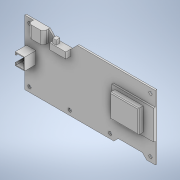
# Autodesk Inventor part: mcu-unit
Saved by Autodesk Inventor 2021 (Build 250183000, 183)
## iProperties
Created: 2024-04-23
Part Number: mcu-unit
Material: Generic
Document SubType Name: Modeling
Designer: Toby
Density: 1 g/cm^3
Appearance: Default
Author: Toby
Autodesk Inventor part; units mm, degrees
ref_plane "YZ Plane" through (0, 0, 0) normal (1, 0, 0) x (0, 1, 0)
ref_plane "XZ Plane" through (0, 0, 0) normal (0, 1, 0) x (-1, 0, 0)
ref_plane "XY Plane" through (0, 0, 0) normal (0, 0, 1) x (1, 0, 0)
sketch "Sketch1" plane through (0, 0, 0) normal (0, 0, 1) x (1, 0, 0)
  line L0 (-40.5, 20) -> (40.5, 20)
  line L1 (40.5, 20) -> (40.5, -20)
  line L2 (40.5, -20) -> (-40.5, -20)
  line L3 (-40.5, -20) -> (-40.5, 20)
  point P0 (0, 0)
  dimension "d0" = 81
  dimension "d1" = 40
  dimension "d2" = 20
  dimension "d3" = 40.5
  constraints: 8 end point, 2 parallel, 1 horizontal, 1 perpendicular
  measures "d0" distance of L0.start L0.end
  measures "d1" distance of L0.end L1.end
  measures "d2" distance from line of point (0, 0) L0
  measures "d3" distance from line of L1 point (0, 0)
extrude "Extrusion1" add sketch "Sketch1" along normal blind 1
sketch "Sketch2" plane through (0, 0, 1) normal (0, 0, 1) x (1, 0, 0)
  line L0 (40.5, 20) -> (-40.5, 20) projected
  line L1 (-21.8, 20) -> (-11.7, 20)
  line L2 (-11.7, 20) -> (-11.7, 16.1)
  line L3 (-11.7, 16.1) -> (-21.8, 16.1)
  line L4 (-21.8, 16.1) -> (-21.8, 20)
  line L5 (-40.5, 20) -> (-40.5, -20) projected
  point P0 (0, 0)
  dimension "d6" = 18.7
  dimension "d7" = 28.8
  dimension "d8" = 3.9
  constraints: 8 end point, 2 parallel, 1 horizontal, 1 perpendicular, 1 point on line
  measures "d6" distance between parallel lines of L5 L4
  measures "d7" distance between parallel lines of L5 L2
  measures "d8" distance between parallel lines of L3 L0
extrude "Extrusion2" cut sketch "Sketch2" against normal blind 1
chamfer "Chamfer1" distance 3.88 angle 45 2 edges at (-21.8, 20, 0.5) (-11.7, 20, 0.5)
sketch "Sketch3" plane through (0, 0, 1) normal (0, 0, 1) x (1, 0, 0)
  line L0 (-25.68, 20) -> (-40.5, 20) projected
  line L1 (-35.04, 20) -> (-25.77, 20)
  line L2 (-25.77, 20) -> (-25.77, 12.38)
  line L3 (-25.77, 12.38) -> (-35.04, 12.38)
  line L4 (-35.04, 12.38) -> (-35.04, 20)
  line L5 (-40.5, 20) -> (-40.5, -20) projected
  point P0 (0, 0)
  dimension "d14" = 5.46
  dimension "d15" = 14.73
  dimension "d16" = 7.62
  constraints: 8 end point, 2 parallel, 1 horizontal, 1 perpendicular, 1 point on line
  measures "d14" distance between parallel lines of L5 L4
  measures "d15" distance between parallel lines of L5 L2
  measures "d16" distance of L3.end L1.start
extrude "Extrusion3" add sketch "Sketch3" along normal blind 3.2
fillet "Fillet1" radius 2 2 edges at (-35.04, 16.19, 4.2) (-25.77, 16.19, 4.2)
sketch "Sketch4" plane through (0, 0, 1) normal (0, 0, 1) x (1, 0, 0)
  line L0 (-11.7, 16.1) -> (-21.8, 16.1) projected
  line L1 (-21.8, 16.1) -> (-11.8, 16.1)
  line L2 (-11.8, 16.1) -> (-11.8, 12.3)
  line L3 (-11.8, 12.3) -> (-21.8, 12.3)
  line L4 (-21.8, 12.3) -> (-21.8, 16.1)
  point P0 (0, 0)
  dimension "d20" = 3.8
  dimension "d21" = 10
  constraints: 8 end point, 2 parallel, 1 horizontal, 1 perpendicular
  measures "d20" distance of L1.end L2.end
  measures "d21" distance between parallel lines of L4 L2
extrude "Extrusion4" add sketch "Sketch4" along normal blind 3.2
sketch "Sketch5" plane through (-21.8, 16.1, 0) normal (0, 1, 0) x (1, 0, 0)
  line L0 (1.2, -3.6) -> (3.4, -3.6)
  line L1 (3.4, -3.6) -> (3.4, -1.2)
  line L2 (3.4, -1.2) -> (1.2, -1.2)
  line L3 (1.2, -1.2) -> (1.2, -3.6)
  line L4 (10, -4.2) -> (0, -4.2) projected
  line L5 (0, -1) -> (0, -4.2) projected
  point P0 (21.8, 0)
  dimension "d24" = 0.6
  dimension "d25" = 1.2
  dimension "d26" = 2.4
  dimension "d27" = 2.2
  constraints: 8 end point, 2 parallel, 1 horizontal, 1 perpendicular
  measures "d24" distance between parallel lines of L4 L0
  measures "d25" distance between parallel lines of L3 L5
  measures "d26" distance of L0.end L1.end
  measures "d27" distance between parallel lines of L3 L1
extrude "Extrusion5" add sketch "Sketch5" along normal blind 2.8
sketch "Sketch6" plane through (0, 0, 1) normal (0, 0, 1) x (1, 0, 0)
  line L0 (-40.5, 20) -> (-40.5, -20) projected
  line L1 (-40.5, -20) -> (40.5, -20) projected
  point P0 (0, 0)
  point P1 (-37.5, -17)
  point P2 (-12.5, -17)
  point P3 (12.5, -17)
  point P4 (37.5, -17)
  dimension "d30" = 3
  dimension "d31" = 28
  dimension "d32" = 53
  dimension "d33" = 78
  dimension "d34" = 3
  dimension "d35" = 3
  dimension "d36" = 3
  dimension "d37" = 3
  measures "d30" distance from line of L0 point (-37.5, -17)
  measures "d31" distance from line of L0 point (-12.5, -17)
  measures "d32" distance from line of L0 point (12.5, -17)
  measures "d33" distance from line of L0 point (37.5, -17)
  measures "d34" distance from line of L1 point (-37.5, -17)
  measures "d35" distance from line of L1 point (-12.5, -17)
  measures "d36" distance from line of L1 point (12.5, -17)
  measures "d37" distance from line of L1 point (37.5, -17)
hole "Hole1" at (-37.5, -17, 1) at (-12.5, -17, 1) at (12.5, -17, 1) at (37.5, -17, 1) direction (0, 0, -1) diameter 2 depth 4 tip angle 118
sketch "Sketch7" plane through (0, 0, 1) normal (0, 0, 1) x (1, 0, 0)
  line L0 (-40.5, 20) -> (-40.5, -20) projected
  line L1 (-40.5, -20) -> (40.5, -20) projected
  point P0 (0, 0)
  point P1 (-37.5, 17)
  point P2 (37.5, 17)
  dimension "d45" = 3
  dimension "d46" = 37
  dimension "d47" = 78
  dimension "d48" = 37
  measures "d45" distance from line of L0 point (-37.5, 17)
  measures "d46" distance from line of L1 point (-37.5, 17)
  measures "d47" distance from line of L0 point (37.5, 17)
  measures "d48" distance from line of L1 point (37.5, 17)
hole "Hole2" at (-37.5, 17, 1) at (37.5, 17, 1) direction (0, 0, -1) diameter 2 depth 4 tip angle 118
sketch "Sketch8" plane through (0, 0, 1) normal (0, 0, 1) x (1, 0, 0)
  line L0 (-40.5, -20) -> (40.5, -20) projected
  line L1 (17.5, -20) -> (32.5, -20)
  line L2 (32.5, -20) -> (32.5, -17.3)
  line L3 (32.5, -17.3) -> (17.5, -17.3)
  line L4 (17.5, -17.3) -> (17.5, -20)
  line L5 (-40.5, 20) -> (-40.5, -20) projected
  point P0 (0, 0)
  dimension "d56" = 58
  dimension "d57" = 73
  dimension "d58" = 2.7
  constraints: 8 end point, 2 parallel, 1 horizontal, 1 perpendicular, 1 point on line
  measures "d56" distance between parallel lines of L5 L4
  measures "d57" distance between parallel lines of L5 L2
  measures "d58" distance between parallel lines of L0 L3
extrude "Extrusion6" cut sketch "Sketch8" against normal blind 2
chamfer "Chamfer2" distance 2.7 angle 45 2 edges at (17.5, -20, 0.5) (32.5, -20, 0.5)
sketch "Sketch9" plane through (0, 0, 1) normal (0, 0, 1) x (1, 0, 0)
  line L0 (-39.36, 4.4) -> (-33.5, 4.4)
  line L1 (-33.5, 4.4) -> (-33.5, -3.1)
  line L2 (-33.5, -3.1) -> (-39.36, -3.1)
  line L3 (-39.36, -3.1) -> (-39.36, 4.4)
  line L4 (-40.5, 20) -> (-40.5, -20) projected
  line L5 (-40.5, -20) -> (14.8, -20) projected
  line L6 (-38.86, 3.9) -> (-34, 3.9)
  line L7 (-34, 3.9) -> (-34, -2.6)
  line L8 (-34, -2.6) -> (-38.86, -2.6)
  line L9 (-38.86, -2.6) -> (-38.86, 3.9)
  line L10 (-39.36, 2.7) -> (-38.86, 2.7)
  line L11 (-38.86, 2.7) -> (-38.86, -1.4)
  line L12 (-38.86, -1.4) -> (-39.36, -1.4)
  line L13 (-39.36, -1.4) -> (-39.36, 2.7)
  point P0 (0, 0)
  dimension "d64" = 1.14
  dimension "d65" = 7
  dimension "d66" = 16.9
  dimension "d67" = 24.4
  dimension "d68" = 0.5
  dimension "d69" = 0.5
  dimension "d70" = 0.5
  dimension "d71" = 0.5
  dimension "d72" = 1.2
  dimension "d73" = 1.2
  constraints: 24 end point, 6 parallel, 3 horizontal, 3 perpendicular, 2 point on line
  measures "d64" distance between parallel lines of L4 L3
  measures "d65" distance between parallel lines of L1 L4
  measures "d66" distance between parallel lines of L5 L2
  measures "d67" distance between parallel lines of L5 L0
  measures "d68" distance between parallel lines of L0 L6
  measures "d69" distance between parallel lines of L2 L8
  measures "d70" distance between parallel lines of L3 L9
  measures "d71" distance between parallel lines of L1 L7
  measures "d72" distance between parallel lines of L10 L6
  measures "d73" distance between parallel lines of L8 L12
extrude "Extrusion7" add sketch "Sketch9" along normal blind 7 contours L0 L1 L2 L3 L12 L9 L8 L7 L6 L10
sketch "Sketch10" plane through (0, 0, 1) normal (0, 0, 1) x (1, 0, 0)
  line L0 (-36.9032, 2.5042) -> (-36.1235, 2.5042)
  line L1 (-36.1235, 2.5042) -> (-36.1235, 2.0109)
  line L2 (-36.1235, 2.0109) -> (-36.9032, 2.0109)
  line L3 (-36.9032, 2.0109) -> (-36.9032, 2.5042)
  line L4 (-36.9032, -0.8534) -> (-36.1235, -0.8534)
  line L5 (-36.1235, -0.8534) -> (-36.1235, -1.3626)
  line L6 (-36.1235, -1.3626) -> (-36.9032, -1.3626)
  line L7 (-36.9032, -1.3626) -> (-36.9032, -0.8534)
  point P0 (0, 0)
  constraints: 16 end point, 4 parallel, 2 horizontal, 2 perpendicular, 2 point on line
extrude "Extrusion8" add sketch "Sketch10" along normal blind 5
sketch "Sketch11" plane through (0, 0, 1) normal (0, 0, 1) x (1, 0, 0)
  line L0 (40.5, -20) -> (40.5, 20) projected
  line L1 (40.5, 11) -> (14.5, 11)
  line L2 (14.5, 11) -> (14.5, -7.2)
  line L3 (14.5, -7.2) -> (40.5, -7.2)
  line L4 (40.5, -7.2) -> (40.5, 11)
  line L5 (-40.5, 20) -> (-40.5, -20) projected
  line L6 (40.5, 20) -> (-7.82, 20) projected
  point P0 (0, 0)
  dimension "d78" = 55
  dimension "d79" = 9
  dimension "d80" = 18.2
  constraints: 8 end point, 2 parallel, 1 horizontal, 1 perpendicular, 1 point on line
  measures "d78" distance between parallel lines of L5 L2
  measures "d79" distance between parallel lines of L6 L1
  measures "d80" distance of L1.end L2.end
extrude "Extrusion9" add sketch "Sketch11" along normal blind 1
sketch "Sketch12" plane through (0, 0, 2) normal (0, 0, 1) x (1, 0, 0)
  line L0 (16.5, 9) -> (34, 9)
  line L1 (34, 9) -> (34, -5.2)
  line L2 (34, -5.2) -> (16.5, -5.2)
  line L3 (16.5, -5.2) -> (16.5, 9)
  line L4 (40.5, 11) -> (14.5, 11) projected
  line L5 (14.5, -7.2) -> (40.5, -7.2) projected
  line L6 (14.5, 11) -> (14.5, -7.2) projected
  line L7 (40.5, -7.2) -> (40.5, 11) projected
  point P0 (0, 0)
  dimension "d83" = 2
  dimension "d84" = 2
  dimension "d85" = 2
  dimension "d86" = 6.5
  constraints: 8 end point, 2 parallel, 1 horizontal, 1 perpendicular
  measures "d83" distance between parallel lines of L0 L4
  measures "d84" distance between parallel lines of L5 L2
  measures "d85" distance between parallel lines of L6 L3
  measures "d86" distance between parallel lines of L7 L1
extrude "Extrusion10" add sketch "Sketch12" along normal blind 3 contours L0 L1 L2 L3
fillet "Fillet2" radius 0.5 4 edges at (25.25, 9, 5) (16.5, 1.9, 5) (25.25, -5.2, 5) (34, 1.9, 5)
sketch "Sketch13" plane through (0, 0, 0) normal (0, 0, -1) x (-1, 0, 0)
  line L0 (-4.4, -16.1) -> (4.4, -16.1)
  line L1 (4.4, -16.1) -> (4.4, -19.4)
  line L2 (4.4, -19.4) -> (-4.4, -19.4)
  line L3 (-4.4, -19.4) -> (-4.4, -16.1)
  line L4 (40.5, 20) -> (40.5, -20) projected
  line L5 (40.5, -20) -> (-14.8, -20) projected
  point P0 (0, 0)
  dimension "d90" = 36.1
  dimension "d91" = 44.9
  dimension "d92" = 0.6
  dimension "d93" = 3.9
  constraints: 8 end point, 2 parallel, 1 horizontal, 1 perpendicular
  measures "d90" distance between parallel lines of L4 L1
  measures "d91" distance between parallel lines of L4 L3
  measures "d92" distance between parallel lines of L5 L2
  measures "d93" distance between parallel lines of L5 L0
extrude "Extrusion11" add sketch "Sketch13" along normal blind 6
fillet "Fillet3" radius 1.28 4 edges at (4.4, -16.1, -3) (4.4, -19.4, -3) (-4.4, -16.1, -3) (-4.4, -19.4, -3)
sketch "Sketch14" plane through (0, 0, 0) normal (0, 0, -1) x (-1, 0, 0)
  line L0 (-32.5, -2.3) -> (-17.3, -2.3)
  line L1 (-17.3, -2.3) -> (-17.3, -17.3)
  line L2 (-17.3, -17.3) -> (-32.5, -17.3)
  line L3 (-32.5, -17.3) -> (-32.5, -2.3)
  line L4 (40.5, 20) -> (40.5, -20) projected
  line L5 (-32.5, -17.3) -> (-17.5, -17.3) projected
  point P0 (0, 0)
  dimension "d97" = 57.8
  dimension "d98" = 73
  dimension "d99" = 15
  constraints: 8 end point, 2 parallel, 1 collinear, 1 horizontal, 1 perpendicular
  measures "d97" distance between parallel lines of L4 L1
  measures "d98" distance between parallel lines of L4 L3
  measures "d99" distance of L2.end L0.start
extrude "Extrusion12" add sketch "Sketch14" along normal blind 2.2
body "Solid1"
